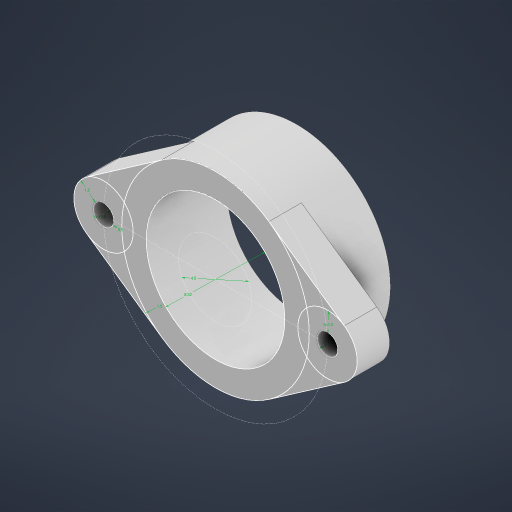
# Autodesk Inventor part: motorauxiliary
Saved by Autodesk Inventor 2023.4 (Build 274418000, 418)
## iProperties
Created: 2024-12-07
Part Number: motorauxiliary
Material: 一般
Document SubType Name: Modeling
Designer: IshiiLabHonda
Density: 1 g/cm^3
Appearance: 既定
Author: IshiiLabHonda
Autodesk Inventor part; units mm, degrees
ref_plane "YZ Plane" through (0, 0, 0) normal (1, 0, 0) x (0, 1, 0)
ref_plane "XZ Plane" through (0, 0, 0) normal (0, 1, 0) x (-1, 0, 0)
ref_plane "XY Plane" through (0, 0, 0) normal (0, 0, 1) x (1, 0, 0)
sketch "スケッチ1" plane through (0, 0, 0) normal (0, 0, 1) x (1, 0, 0)
  circle A0 centre (0, 0) radius 2.25 construction
  circle A1 centre (0, 0) radius 4.26
  circle A2 centre (0, 0) radius 5.76
  circle A3 centre (-6.885, 0) radius 0.625
  circle A4 centre (6.885, 0) radius 0.625
  line L0 (-6.885, 0) -> (6.885, 0) construction
  circle A5 centre (0, 0) radius 6.885 construction
  circle A6 centre (-6.885, 0) radius 1.825
  circle A7 centre (6.885, 0) radius 1.825
  line L1 (-7.928, 1.4976) -> (-3.292, 4.7265)
  line L2 (-7.928, -1.4976) -> (-3.292, -4.7265)
  line L3 (7.928, -1.4976) -> (3.292, -4.7265)
  line L4 (3.292, 4.7265) -> (7.928, 1.4976)
  point P0 (5.61, -1.3058)
  point P1 (5.61, 1.3058)
  point P2 (-5.61, 1.3058)
  point P3 (-5.61, -1.3058)
  dimension "d2" = 4.5
  dimension "d3" = 8.52
  dimension "d4" = 1.5
  dimension "d5" = 1.25
  dimension "d6" = 1.25
  dimension "d7" = 1.2
  dimension "d8" = 1.2
  dimension "d9" = 0.5
  constraints: 10 end point, 10 point on circle, 8 centre point, 8 tangent, 6 coincident, 2 midpoint, 1 horizontal
  measures "d2" diameter of A0
  measures "d3" diameter of A1
  measures "d4" radial gap between concentric circles of A2 A1
  measures "d5" diameter of A4
  measures "d6" diameter of A3
  measures "d7" radial gap between concentric circles of A6 A3
  measures "d8" radial gap between concentric circles of A7 A4
extrude "押し出し1" add sketch "スケッチ1" against normal blind 5 contours A2 A7 A6
extrude "押し出し2" add sketch "スケッチ1" against normal blind 5 contours A2 A7 | A6 A2 picked at (5.525, -0.2154) picked at (-5.5155, 0)
extrude "押し出し3" add sketch "スケッチ1" against normal blind 2 contours A2 A6 L1 | A2 A6 | A2 L2 A6 picked at (-5.9611, -0.7529)
extrude "押し出し4" add sketch "スケッチ1" against normal blind 2 contours L4 A7 A2 | A7 A2 | A7 L3 A2 picked at (6.055, 0.9838)
equation "\"d6\" = d5"
equation "\"d8\" = d7"
